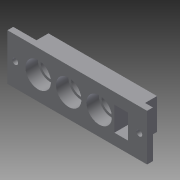
# Autodesk Inventor part: switch and led mount
Saved by Autodesk Inventor 2014 SP1 (Build 180222100, 222)
## iProperties
Created: 2017-06-15
Part Number: switch and led mount
Material: Generic
Document SubType Name: Modeling
Designer: kteo17
Density: 1 g/cm^3
Appearance: Default
Author: kteo17
Autodesk Inventor part; units mm, degrees
ref_plane "YZ Plane" through (0, 0, 0) normal (1, 0, 0) x (0, 1, 0)
ref_plane "XZ Plane" through (0, 0, 0) normal (0, 1, 0) x (-1, 0, 0)
ref_plane "XY Plane" through (0, 0, 0) normal (0, 0, 1) x (1, 0, 0)
sketch "Sketch1" plane through (0, 0, 0) normal (0, 0, 1) x (1, 0, 0)
  line L0 (0, 0) -> (44.45, 0)
  line L1 (44.45, 0) -> (44.45, 12.7)
  line L2 (44.45, 12.7) -> (0, 12.7)
  line L3 (0, 12.7) -> (0, 0)
  dimension "d0" = 44.45
  dimension "d1" = 12.7
  constraints: 8 end point, 2 parallel, 1 horizontal, 1 perpendicular
  measures "d0" distance of L1.end L2.end
  measures "d1" distance of L0.end L1.end
extrude "Extrusion1" add sketch "Sketch1" along normal blind 12.7
sketch "Sketch2" plane through (0, 0, 12.7) normal (0, 0, 1) x (1, 0, 0)
  line L0 (0, 0) -> (44.45, 0) projected
  line L1 (44.45, 0) -> (44.45, 12.7) projected
  line L2 (44.45, 12.7) -> (0, 12.7) projected
  line L3 (0, 12.7) -> (0, 0) projected
  line L4 (-6.35, 15.8432) -> (50.8, 15.8432)
  line L5 (50.8, 15.8432) -> (50.8, -3.175)
  line L6 (50.8, -3.175) -> (-6.35, -3.175)
  line L7 (-6.35, -3.175) -> (-6.35, 15.8432)
  constraints: 8 end point, 2 parallel, 1 horizontal, 1 perpendicular
extrude "Extrusion2" add sketch "Sketch2" against normal blind 2.3813
sketch "Sketch3" plane through (0, 0, 0) normal (0, 0, -1) x (-1, 0, 0)
  line L0 (-44.45, 12.7) -> (0, 12.7) projected
  line L1 (-44.45, 0) -> (-44.45, 12.7) projected
  line L2 (-43.0022, 11.303) -> (-37.4142, 11.303)
  line L3 (-37.4142, 11.303) -> (-37.4142, 1.397)
  line L4 (-37.4142, 1.397) -> (-43.0022, 1.397)
  line L5 (-43.0022, 1.397) -> (-43.0022, 11.303)
  line L6 (0, 12.7) -> (0, 0) projected
  line L7 (-59.9726, 12.7) -> (-59.9726, 0)
  dimension "d13" = 5.588
  dimension "d14" = 1.4478
  dimension "d16" = 9.906
  dimension "d95" = 1.397
  constraints: 10 end point, 3 parallel, 1 horizontal, 1 perpendicular
  measures "d13" distance of L3.end L4.end
  measures "d14" distance between parallel lines of L1 L5
  measures "d16" distance of L2.end L3.end
  measures "d95" distance between parallel lines of L0 L2
extrude "Extrusion3" cut sketch "Sketch3" against normal blind 11.1125
sketch "Sketch5" plane through (0, 0, 10.3188) normal (0, 0, -1) x (-1, 0, 0)
  circle A0 centre (-47.625, 6.3341) radius 1.1906
  circle A1 centre (3.175, 6.35) radius 1.1906
  dimension "d25" = 2.3813
  dimension "d26" = 2.3813
  constraints: 2 centre point
  measures "d25" diameter of A0
  measures "d26" diameter of A1
extrude "Extrusion5" cut sketch "Sketch5" against normal blind 2.3813
sketch "Sketch8" plane through (0, 0, 0) normal (0, 0, -1) x (-1, 0, 0)
  circle A0 centre (-6.2357, 6.35) radius 4.1275
  circle A1 centre (-18.7071, 6.35) radius 4.1275
  circle A2 centre (-31.1785, 6.35) radius 4.1275
  circle A3 centre (-18.7071, 6.35) radius 5.207
  circle A4 centre (-31.1785, 6.35) radius 5.207
  circle A5 centre (-6.2357, 6.35) radius 5.207
  dimension "d47" = 8.255
  dimension "d48" = 8.255
  dimension "d49" = 8.255
  dimension "d53" = 10.414
  dimension "d77" = 10.414
  dimension "d78" = 10.414
  constraints: 6 centre point, 3 coincident
  measures "d47" diameter of A0
  measures "d48" diameter of A1
  measures "d49" diameter of A2
  measures "d53" diameter of A3
  measures "d77" diameter of A5
  measures "d78" diameter of A4
extrude "Extrusion8" cut sketch "Sketch8" against normal blind 11.1125
sketch "Sketch9" plane through (0, 0, 0) normal (0, 0, -1) x (-1, 0, 0)
  circle A0 centre (-31.1785, 6.35) radius 5.207 projected
  circle A1 centre (-18.7071, 6.35) radius 5.207 projected
  circle A2 centre (-6.2357, 6.35) radius 5.207 projected
  circle A3 centre (-6.2357, 6.35) radius 4.1275
  circle A4 centre (-18.7071, 6.35) radius 4.1275
  circle A5 centre (-31.1785, 6.35) radius 4.1275
  dimension "d56" = 8.255
  dimension "d57" = 8.255
  dimension "d58" = 8.255
  constraints: 3 centre point, 3 coincident
  measures "d56" diameter of A3
  measures "d57" diameter of A4
  measures "d58" diameter of A5
extrude "Extrusion9" cut sketch "Sketch9" against normal blind 12.7 contours A3 | A4 | A5
sketch "Sketch10" plane through (0, 0, 0) normal (0, 0, -1) x (-1, 0, 0)
  line L0 (-43.0022, 1.397) -> (-43.0022, 11.303) projected
  line L1 (-43.0022, 11.303) -> (-37.4142, 11.303) projected
  line L2 (-37.4142, 11.303) -> (-37.4142, 1.397) projected
  line L3 (-37.4142, 1.397) -> (-43.0022, 1.397) projected
  circle A0 centre (-31.1785, 6.35) radius 5.207 projected
  circle A1 centre (-18.7071, 6.35) radius 5.207 projected
  circle A2 centre (-6.2357, 6.35) radius 5.207 projected
extrude "Extrusion10" cut sketch "Sketch10" against normal blind 12.7
sketch "Sketch11" plane through (0, 0, 0) normal (0, 0, -1) x (-1, 0, 0)
  line L0 (-43.0022, 1.397) -> (-43.0022, 11.303) projected
  line L1 (-43.0022, 11.303) -> (-37.4142, 11.303) projected
  line L2 (-37.4142, 11.303) -> (-37.4142, 1.397) projected
  line L3 (-37.4142, 1.397) -> (-43.0022, 1.397) projected
  circle A0 centre (-31.1785, 6.35) radius 5.207 projected
  circle A1 centre (-18.7071, 6.35) radius 5.207 projected
  circle A2 centre (-6.2357, 6.35) radius 5.207 projected
  circle A3 centre (-6.2357, 6.35) radius 4.1275
  circle A4 centre (-18.7071, 6.35) radius 4.1275
  circle A5 centre (-31.1785, 6.35) radius 4.1275
  line L4 (-43.0022, 9.525) -> (-37.4142, 9.525)
  line L5 (-43.0022, 3.175) -> (-37.4142, 3.175)
  dimension "d63" = 8.255
  constraints: 4 end point, 4 point on line, 3 centre point, 3 coincident, 1 perpendicular
  measures "d63" diameter of A3
extrude "Extrusion11" add sketch "Sketch11" against normal blind 7.62 contours L0 L5 L2 L3 | L0 L1 L2 L4 | A0 | A1 | A2
sketch "Sketch12" plane through (0, 0, 12.7) normal (0, 0, 1) x (1, 0, 0)
  line L0 (43.0022, 1.397) -> (37.4142, 1.397) projected
  line L1 (37.4142, 1.397) -> (37.4142, 11.303) projected
  line L2 (37.4142, 11.303) -> (43.0022, 11.303) projected
  line L3 (43.0022, 11.303) -> (43.0022, 1.397) projected
  point P0 (0, 0)
extrude "Extrusion12" cut sketch "Sketch12" against normal blind 9.525
sketch "Sketch15" plane through (0, 0, 0) normal (0, 0, -1) x (-1, 0, 0)
  circle A0 centre (-6.2357, 6.35) radius 4.1275 projected
  circle A1 centre (-31.1785, 6.35) radius 4.1275 projected
  circle A2 centre (-18.7071, 6.35) radius 4.1275 projected
  line L0 (0, 0) -> (-44.45, 0) projected
  line L1 (0, 12.7) -> (0, 0) projected
  line L2 (-44.45, 12.7) -> (0, 12.7) projected
  line L3 (-44.45, 0) -> (-44.45, 12.7) projected
  line L4 (-43.0022, 3.175) -> (-43.0022, 9.525) projected
  line L5 (-43.0022, 9.525) -> (-37.4142, 9.525) projected
  line L6 (-37.4142, 9.525) -> (-37.4142, 3.175) projected
  line L7 (-37.4142, 3.175) -> (-43.0022, 3.175) projected
extrude "Extrusion15" cut sketch "Sketch15" against normal blind 2.286
sketch "Sketch16" plane through (0, 0, 12.7) normal (0, 0, 1) x (1, 0, 0)
  line L0 (37.4142, 1.397) -> (37.4142, 11.303) projected
  line L1 (43.0022, 11.303) -> (43.0022, 1.397) projected
  line L2 (37.4142, 11.303) -> (43.0022, 9.525)
  line L3 (37.4142, 1.397) -> (43.0022, 3.1742)
  line L4 (43.0022, 3.1742) -> (43.0022, 9.525)
  line L5 (37.4142, 1.397) -> (37.4142, 11.303)
  point P0 (0, 0)
  constraints: 8 end point, 2 collinear, 1 point on line
extrude "Extrusion16" cut sketch "Sketch16" against normal blind 25.4
body "Solid1"
